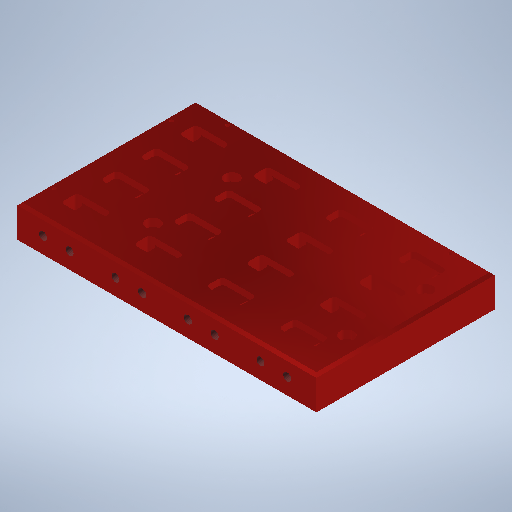
# Autodesk Inventor part: Chuck - 16-pocket
Saved by Autodesk Inventor 2025 (Build 290162000, 162)
## iProperties
Created: 2014-01-09
Part Number: Chuck - 16-pocket
Material: Aluminum, Anodized Red
Document SubType Name: Modeling
Designer: Caleb Fangmeier
Density: 2.7 g/cm^3
Project: CMS ETL
Mass: 2699.72 g
Surface Area: 1115.91 cm^2
Volume: 999.896 cm^3
Appearance: Anodized - Red
Author: Frank Meier
Autodesk Inventor part; units mm, degrees
ref_plane "YZ Plane" through (0, 0, 0) normal (1, 0, 0) x (0, 1, 0)
ref_plane "XZ Plane" through (0, 0, 0) normal (0, 1, 0) x (-1, 0, 0)
ref_plane "XY Plane" through (0, 0, 0) normal (0, 0, 1) x (1, 0, 0)
sketch "Skizze1" plane through (0, 0, 0) normal (0, 0, 1) x (1, 0, 0)
  line L0 (-117.5, -70) -> (117.5, -70)
  line L1 (117.5, -70) -> (117.5, 70)
  line L2 (117.5, 70) -> (-117.5, 70)
  line L3 (-117.5, 70) -> (-117.5, -70)
  line L4 (-117.5, -70) -> (117.5, 70) construction
  line L5 (117.5, -70) -> (-117.5, 70) construction
  point P0 (0, 0)
  dimension "d0" = 235
  dimension "d2" = 140
  constraints: 12 end point, 2 midpoint, 2 parallel, 1 horizontal, 1 perpendicular
  measures "d0" distance of L1.end L2.end
  measures "d2" distance of L0.end L1.end
extrude "Extrusion1" add sketch "Skizze1" along normal blind 25.4
chamfer "Fase1" distance 2 angle 45 4 edges at (0, -70, 25.4) (-117.5, 0, 25.4) (0, 70, 25.4) (117.5, 0, 25.4)
sketch "Alignment Holes" plane through (0, 0, 25.4) normal (0, 0, 1) x (1, 0, 0)
  line L0 (117.5, 70) -> (-117.5, 70) projected
  line L1 (117.5, -70) -> (117.5, 70) projected
  line L2 (-117.5, 70) -> (-117.5, -70) projected
  line L3 (-117.5, -70) -> (117.5, -70) projected
  point P0 (-112.5, 46)
  point P1 (-112.5, -46)
  point P2 (-87.5, 65)
  point P3 (87.5, 65)
  dimension "d153" = 24
  dimension "d154" = 24
  dimension "d155" = 5
  dimension "d158" = 5
  dimension "d159" = 5
  dimension "d160" = 30
  dimension "d161" = 30
  dimension "d162" = 5
  measures "d153" distance from line of L0 point (-112.5, 46)
  measures "d154" distance from line of L3 point (-112.5, -46)
  measures "d155" distance from line of L2 point (-112.5, -46)
  measures "d158" distance from line of L2 point (-112.5, 46)
  measures "d159" distance from line of L0 point (-87.5, 65)
  measures "d160" distance from line of L2 point (-87.5, 65)
  measures "d161" distance from line of L1 point (87.5, 65)
  measures "d162" distance from line of L0 point (87.5, 65)
hole "Bohrung7" at (-112.5, 46, 25.4) at (-112.5, -46, 25.4) at (-87.5, 65, 25.4) at (87.5, 65, 25.4) direction (0, 0, -1) diameter 3 end through all
sketch "Wells" plane through (0, 0, 25.4) normal (0, 0, 1) x (1, 0, 0)
  line L0 (-97.5, 53) -> (-76.5, 53)
  line L1 (-73.5, 50) -> (-73.5, 43)
  line L2 (-76.5, 40) -> (-97.5, 40)
  line L3 (-100.5, 43) -> (-100.5, 50)
  circle A0 centre (-87.5, 65) radius 1.5 projected
  circle A1 centre (-112.5, 46) radius 1.5 projected
  arc A2 (-97.5, 53) -> (-100.5, 50) centre (-97.5, 50) ccw
  arc A3 (-73.5, 50) -> (-76.5, 53) centre (-76.5, 50) ccw
  arc A4 (-76.5, 40) -> (-73.5, 43) centre (-76.5, 43) ccw
  arc A5 (-100.5, 43) -> (-97.5, 40) centre (-97.5, 43) ccw
  arc A6 (-40.5, 53) -> (-43.5, 50) centre (-40.5, 50) ccw
  line L4 (-43.5, 43) -> (-43.5, 50)
  arc A7 (-43.5, 43) -> (-40.5, 40) centre (-40.5, 43) ccw
  line L5 (-40.5, 53) -> (-19.5, 53)
  arc A8 (-16.5, 50) -> (-19.5, 53) centre (-19.5, 50) ccw
  line L6 (-16.5, 50) -> (-16.5, 43)
  line L7 (-19.5, 40) -> (-40.5, 40)
  arc A9 (-19.5, 40) -> (-16.5, 43) centre (-19.5, 43) ccw
  arc A10 (16.5, 53) -> (13.5, 50) centre (16.5, 50) ccw
  line L8 (13.5, 43) -> (13.5, 50)
  arc A11 (13.5, 43) -> (16.5, 40) centre (16.5, 43) ccw
  line L9 (16.5, 53) -> (37.5, 53)
  arc A12 (40.5, 50) -> (37.5, 53) centre (37.5, 50) ccw
  line L10 (40.5, 50) -> (40.5, 43)
  line L11 (37.5, 40) -> (16.5, 40)
  arc A13 (37.5, 40) -> (40.5, 43) centre (37.5, 43) ccw
  arc A14 (73.5, 53) -> (70.5, 50) centre (73.5, 50) ccw
  line L12 (70.5, 43) -> (70.5, 50)
  arc A15 (70.5, 43) -> (73.5, 40) centre (73.5, 43) ccw
  line L13 (73.5, 53) -> (94.5, 53)
  arc A16 (97.5, 50) -> (94.5, 53) centre (94.5, 50) ccw
  line L14 (97.5, 50) -> (97.5, 43)
  line L15 (94.5, 40) -> (73.5, 40)
  arc A17 (94.5, 40) -> (97.5, 43) centre (94.5, 43) ccw
  arc A18 (-97.5, 22) -> (-100.5, 19) centre (-97.5, 19) ccw
  line L16 (-100.5, 12) -> (-100.5, 19)
  arc A19 (-100.5, 12) -> (-97.5, 9) centre (-97.5, 12) ccw
  line L17 (-97.5, 22) -> (-76.5, 22)
  arc A20 (-73.5, 19) -> (-76.5, 22) centre (-76.5, 19) ccw
  line L18 (-73.5, 19) -> (-73.5, 12)
  line L19 (-76.5, 9) -> (-97.5, 9)
  arc A21 (-76.5, 9) -> (-73.5, 12) centre (-76.5, 12) ccw
  arc A22 (-40.5, 22) -> (-43.5, 19) centre (-40.5, 19) ccw
  line L20 (-43.5, 12) -> (-43.5, 19)
  arc A23 (-43.5, 12) -> (-40.5, 9) centre (-40.5, 12) ccw
  line L21 (-40.5, 22) -> (-19.5, 22)
  arc A24 (-16.5, 19) -> (-19.5, 22) centre (-19.5, 19) ccw
  line L22 (-16.5, 19) -> (-16.5, 12)
  line L23 (-19.5, 9) -> (-40.5, 9)
  arc A25 (-19.5, 9) -> (-16.5, 12) centre (-19.5, 12) ccw
  arc A26 (16.5, 22) -> (13.5, 19) centre (16.5, 19) ccw
  line L24 (13.5, 12) -> (13.5, 19)
  arc A27 (13.5, 12) -> (16.5, 9) centre (16.5, 12) ccw
  line L25 (16.5, 22) -> (37.5, 22)
  arc A28 (40.5, 19) -> (37.5, 22) centre (37.5, 19) ccw
  line L26 (40.5, 19) -> (40.5, 12)
  line L27 (37.5, 9) -> (16.5, 9)
  arc A29 (37.5, 9) -> (40.5, 12) centre (37.5, 12) ccw
  arc A30 (73.5, 22) -> (70.5, 19) centre (73.5, 19) ccw
  line L28 (70.5, 12) -> (70.5, 19)
  arc A31 (70.5, 12) -> (73.5, 9) centre (73.5, 12) ccw
  line L29 (73.5, 22) -> (94.5, 22)
  arc A32 (97.5, 19) -> (94.5, 22) centre (94.5, 19) ccw
  line L30 (97.5, 19) -> (97.5, 12)
  line L31 (94.5, 9) -> (73.5, 9)
  arc A33 (94.5, 9) -> (97.5, 12) centre (94.5, 12) ccw
  arc A34 (-97.5, -9) -> (-100.5, -12) centre (-97.5, -12) ccw
  line L32 (-100.5, -19) -> (-100.5, -12)
  arc A35 (-100.5, -19) -> (-97.5, -22) centre (-97.5, -19) ccw
  line L33 (-97.5, -9) -> (-76.5, -9)
  arc A36 (-73.5, -12) -> (-76.5, -9) centre (-76.5, -12) ccw
  line L34 (-73.5, -12) -> (-73.5, -19)
  line L35 (-76.5, -22) -> (-97.5, -22)
  arc A37 (-76.5, -22) -> (-73.5, -19) centre (-76.5, -19) ccw
  arc A38 (-40.5, -9) -> (-43.5, -12) centre (-40.5, -12) ccw
  line L36 (-43.5, -19) -> (-43.5, -12)
  arc A39 (-43.5, -19) -> (-40.5, -22) centre (-40.5, -19) ccw
  line L37 (-40.5, -9) -> (-19.5, -9)
  arc A40 (-16.5, -12) -> (-19.5, -9) centre (-19.5, -12) ccw
  line L38 (-16.5, -12) -> (-16.5, -19)
  line L39 (-19.5, -22) -> (-40.5, -22)
  arc A41 (-19.5, -22) -> (-16.5, -19) centre (-19.5, -19) ccw
  arc A42 (16.5, -9) -> (13.5, -12) centre (16.5, -12) ccw
  line L40 (13.5, -19) -> (13.5, -12)
  arc A43 (13.5, -19) -> (16.5, -22) centre (16.5, -19) ccw
  line L41 (16.5, -9) -> (37.5, -9)
  arc A44 (40.5, -12) -> (37.5, -9) centre (37.5, -12) ccw
  line L42 (40.5, -12) -> (40.5, -19)
  line L43 (37.5, -22) -> (16.5, -22)
  arc A45 (37.5, -22) -> (40.5, -19) centre (37.5, -19) ccw
  arc A46 (73.5, -9) -> (70.5, -12) centre (73.5, -12) ccw
  line L44 (70.5, -19) -> (70.5, -12)
  arc A47 (70.5, -19) -> (73.5, -22) centre (73.5, -19) ccw
  line L45 (73.5, -9) -> (94.5, -9)
  arc A48 (97.5, -12) -> (94.5, -9) centre (94.5, -12) ccw
  line L46 (97.5, -12) -> (97.5, -19)
  line L47 (94.5, -22) -> (73.5, -22)
  arc A49 (94.5, -22) -> (97.5, -19) centre (94.5, -19) ccw
  arc A50 (-97.5, -40) -> (-100.5, -43) centre (-97.5, -43) ccw
  line L48 (-100.5, -50) -> (-100.5, -43)
  arc A51 (-100.5, -50) -> (-97.5, -53) centre (-97.5, -50) ccw
  line L49 (-97.5, -40) -> (-76.5, -40)
  arc A52 (-73.5, -43) -> (-76.5, -40) centre (-76.5, -43) ccw
  line L50 (-73.5, -43) -> (-73.5, -50)
  line L51 (-76.5, -53) -> (-97.5, -53)
  arc A53 (-76.5, -53) -> (-73.5, -50) centre (-76.5, -50) ccw
  arc A54 (-40.5, -40) -> (-43.5, -43) centre (-40.5, -43) ccw
  line L52 (-43.5, -50) -> (-43.5, -43)
  arc A55 (-43.5, -50) -> (-40.5, -53) centre (-40.5, -50) ccw
  line L53 (-40.5, -40) -> (-19.5, -40)
  arc A56 (-16.5, -43) -> (-19.5, -40) centre (-19.5, -43) ccw
  line L54 (-16.5, -43) -> (-16.5, -50)
  line L55 (-19.5, -53) -> (-40.5, -53)
  arc A57 (-19.5, -53) -> (-16.5, -50) centre (-19.5, -50) ccw
  arc A58 (16.5, -40) -> (13.5, -43) centre (16.5, -43) ccw
  line L56 (13.5, -50) -> (13.5, -43)
  arc A59 (13.5, -50) -> (16.5, -53) centre (16.5, -50) ccw
  line L57 (16.5, -40) -> (37.5, -40)
  arc A60 (40.5, -43) -> (37.5, -40) centre (37.5, -43) ccw
  line L58 (40.5, -43) -> (40.5, -50)
  line L59 (37.5, -53) -> (16.5, -53)
  arc A61 (37.5, -53) -> (40.5, -50) centre (37.5, -50) ccw
  arc A62 (73.5, -40) -> (70.5, -43) centre (73.5, -43) ccw
  line L60 (70.5, -50) -> (70.5, -43)
  arc A63 (70.5, -50) -> (73.5, -53) centre (73.5, -50) ccw
  line L61 (73.5, -40) -> (94.5, -40)
  arc A64 (97.5, -43) -> (94.5, -40) centre (94.5, -43) ccw
  line L62 (97.5, -43) -> (97.5, -50)
  line L63 (94.5, -53) -> (73.5, -53)
  arc A65 (94.5, -53) -> (97.5, -50) centre (94.5, -50) ccw
  line L64 (117.5, 70) -> (-117.5, 70) projected
  line L65 (-117.5, 70) -> (-117.5, -70) projected
  line L66 (-117.5, -70) -> (117.5, -70) projected
  line L67 (117.5, -70) -> (117.5, 70) projected
  point P0 (0, 0)
  point P1 (-73.5, 40)
  point P2 (-73.5, 53)
  point P3 (-100.5, 40)
  point P4 (-43.5, 40)
  point P5 (-16.5, 53)
  point P6 (-16.5, 40)
  point P7 (13.5, 40)
  point P8 (40.5, 53)
  point P9 (40.5, 40)
  point P10 (70.5, 40)
  point P11 (97.5, 53)
  point P12 (97.5, 40)
  point P13 (-100.5, 9)
  point P14 (-73.5, 22)
  point P15 (-73.5, 9)
  point P16 (-43.5, 9)
  point P17 (-16.5, 22)
  point P18 (-16.5, 9)
  point P19 (13.5, 9)
  point P20 (40.5, 22)
  point P21 (40.5, 9)
  point P22 (70.5, 9)
  point P23 (97.5, 22)
  point P24 (97.5, 9)
  point P25 (-100.5, -22)
  point P26 (-73.5, -9)
  point P27 (-73.5, -22)
  point P28 (-43.5, -22)
  point P29 (-16.5, -9)
  point P30 (-16.5, -22)
  point P31 (13.5, -22)
  point P32 (40.5, -9)
  point P33 (40.5, -22)
  point P34 (70.5, -22)
  point P35 (97.5, -9)
  point P36 (97.5, -22)
  point P37 (-100.5, -53)
  point P38 (-73.5, -40)
  point P39 (-73.5, -53)
  point P40 (-43.5, -53)
  point P41 (-16.5, -40)
  point P42 (-16.5, -53)
  point P43 (13.5, -53)
  point P44 (40.5, -40)
  point P45 (40.5, -53)
  point P46 (70.5, -53)
  point P47 (97.5, -40)
  point P48 (97.5, -53)
  dimension "d259" = 27
  dimension "d260" = 13
  dimension "d266" = 3
  dimension "d269" = 57
  dimension "d272" = 31
  dimension "d476" = 17
  dimension "d477" = 17
  dimension "d478" = 17
  dimension "d479" = 20
  constraints: 128 end point, 128 point on circle, 96 point on line, 64 centre point, 8 tangent, 3 equal radius, 2 collinear, 2 horizontal, 2 parallel, 1 perpendicular, 1 vertical, 343 other
  measures "d259" distance of point (-73.5, 40) point (-100.5, 40)
  measures "d260" distance of point (-73.5, 53) point (-73.5, 40)
  measures "d266" radius of A2
  measures "d269" distance of L3.end L4.end
  measures "d272" distance of L3.end L16.end
  measures "d476" distance between parallel lines of L64 L0
  measures "d477" distance between parallel lines of L65 L3
  measures "d478" distance between parallel lines of L66 L51
  measures "d479" distance between parallel lines of L67 L14
extrude "Extrusion6" cut sketch "Wells" against normal blind 5 contours L0 A3 L1 A4 L2 A5 L3 A2 | L5 A8 L6 A9 L7 A7 L4 A6 | L9 A12 L10 A13 L11 A11 L8 A10 | L13 A16 L14 A17 L15 A15 L12 A14 | L17 A20 L18 A21 L19 A19 L16 A18 | L21 A24 L22 A25 L23 A23 L20 A22 | L25 A28 L26 A29 L27 A27 L24 A26 | L29 A32 L30 A33 L31 A31 L28 A30 | L33 A36 L34 A37 L35 A35 L32 A34 | L37 A40 L38 A41 L39 A39 L36 A38 | L41 A44 L42 A45 L43 A43 L40 A42 | L45 A48 L46 A49 L47 A47 L44 A46 | L49 A52 L50 A53 L51 A51 L48 A50 | L53 A56 L54 A57 L55 A55 L52 A54 | L57 A60 L58 A61 L59 A59 L56 A58 | L61 A64 L62 A65 L63 A63 L60 A62
sketch "Sketch22" plane through (0, 0, 25.4) normal (0, 0, 1) x (1, 0, 0)
  point P0 (0, 0)
  point P1 (102.4, -31)
  point P2 (-50, -31)
  point P3 (-50, 31)
  point P4 (102.4, 31)
  dimension "d383" = 152.4
  dimension "d384" = 31
  dimension "d385" = 62
  dimension "d503" = 50
  constraints: 2 horizontal alignment, 2 vertical alignment
  measures "d383" distance of point (102.4, -31) point (-50, -31)
  measures "d384" vertical distance of point (102.4, -31) point (0, 0)
  measures "d385" distance of point (102.4, -31) point (102.4, 31)
  measures "d503" horizontal distance of point (-50, 31) point (0, 0)
hole "Hole18" at (102.4, -31, 25.4) at (-50, -31, 25.4) at (-50, 31, 25.4) at (102.4, 31, 25.4) direction (0, 0, -1) diameter 6.528 end through all counterbore diameter 11.113 counterbore depth 6.35 clearance for "Socket Head Cap Screw" size "1/4" standard "Ansi Unified Screw Threads"
sketch "Sketch24" plane through (0, 0, 25.4) normal (0, 0, 1) x (1, 0, 0)
  line L0 (-76.5, 40) -> (-97.5, 40) projected
  arc A0 (-76.5, 40) -> (-73.5, 43) centre (-76.5, 43) ccw projected
  line L1 (-73.5, 50) -> (-73.5, 43) projected
  arc A1 (-73.5, 50) -> (-76.5, 53) centre (-76.5, 50) ccw projected
  line L2 (-97.5, 53) -> (-76.5, 53) projected
  arc A2 (-97.5, 53) -> (-100.5, 50) centre (-97.5, 50) ccw projected
  line L3 (-100.5, 43) -> (-100.5, 50) projected
  arc A3 (-100.5, 43) -> (-97.5, 40) centre (-97.5, 43) ccw projected
  line L4 (-76.5, 39.25) -> (-97.5, 39.25)
  line L5 (-101.25, 43) -> (-101.25, 50)
  line L6 (-97.5, 53.75) -> (-76.5, 53.75)
  line L7 (-72.75, 50) -> (-72.75, 43)
  line L8 (-76.5, 37.75) -> (-97.5, 37.75)
  line L9 (-102.75, 43) -> (-102.75, 50)
  line L10 (-97.5, 55.25) -> (-76.5, 55.25)
  line L11 (-71.25, 50) -> (-71.25, 43)
  arc A4 (-97.5, 53.75) -> (-101.25, 50) centre (-97.5, 50) ccw
  arc A5 (-97.5, 55.25) -> (-102.75, 50) centre (-97.5, 50) ccw
  arc A6 (-101.25, 43) -> (-97.5, 39.25) centre (-97.5, 43) ccw
  arc A7 (-76.5, 39.25) -> (-72.75, 43) centre (-76.5, 43) ccw
  arc A8 (-72.75, 50) -> (-76.5, 53.75) centre (-76.5, 50) ccw
  arc A9 (-102.75, 43) -> (-97.5, 37.75) centre (-97.5, 43) ccw
  arc A10 (-76.5, 37.75) -> (-71.25, 43) centre (-76.5, 43) ccw
  arc A11 (-71.25, 50) -> (-76.5, 55.25) centre (-76.5, 50) ccw
  arc A12 (-19.5, 39.25) -> (-15.75, 43) centre (-19.5, 43) ccw
  arc A13 (-19.5, 37.75) -> (-14.25, 43) centre (-19.5, 43) ccw
  arc A14 (-15.75, 50) -> (-19.5, 53.75) centre (-19.5, 50) ccw
  arc A15 (-14.25, 50) -> (-19.5, 55.25) centre (-19.5, 50) ccw
  line L12 (-14.25, 50) -> (-14.25, 43)
  line L13 (-15.75, 50) -> (-15.75, 43)
  line L14 (-19.5, 37.75) -> (-40.5, 37.75)
  line L15 (-19.5, 39.25) -> (-40.5, 39.25)
  line L16 (-40.5, 55.25) -> (-19.5, 55.25)
  line L17 (-40.5, 53.75) -> (-19.5, 53.75)
  line L18 (-44.25, 43) -> (-44.25, 50)
  line L19 (-45.75, 43) -> (-45.75, 50)
  arc A16 (-44.25, 43) -> (-40.5, 39.25) centre (-40.5, 43) ccw
  arc A17 (-45.75, 43) -> (-40.5, 37.75) centre (-40.5, 43) ccw
  arc A18 (-40.5, 53.75) -> (-44.25, 50) centre (-40.5, 50) ccw
  arc A19 (-40.5, 55.25) -> (-45.75, 50) centre (-40.5, 50) ccw
  arc A20 (37.5, 39.25) -> (41.25, 43) centre (37.5, 43) ccw
  arc A21 (37.5, 37.75) -> (42.75, 43) centre (37.5, 43) ccw
  arc A22 (41.25, 50) -> (37.5, 53.75) centre (37.5, 50) ccw
  arc A23 (42.75, 50) -> (37.5, 55.25) centre (37.5, 50) ccw
  line L20 (42.75, 50) -> (42.75, 43)
  line L21 (41.25, 50) -> (41.25, 43)
  line L22 (37.5, 37.75) -> (16.5, 37.75)
  line L23 (37.5, 39.25) -> (16.5, 39.25)
  line L24 (16.5, 55.25) -> (37.5, 55.25)
  line L25 (16.5, 53.75) -> (37.5, 53.75)
  line L26 (12.75, 43) -> (12.75, 50)
  line L27 (11.25, 43) -> (11.25, 50)
  arc A24 (12.75, 43) -> (16.5, 39.25) centre (16.5, 43) ccw
  arc A25 (11.25, 43) -> (16.5, 37.75) centre (16.5, 43) ccw
  arc A26 (16.5, 53.75) -> (12.75, 50) centre (16.5, 50) ccw
  arc A27 (16.5, 55.25) -> (11.25, 50) centre (16.5, 50) ccw
  arc A28 (94.5, 39.25) -> (98.25, 43) centre (94.5, 43) ccw
  arc A29 (94.5, 37.75) -> (99.75, 43) centre (94.5, 43) ccw
  arc A30 (98.25, 50) -> (94.5, 53.75) centre (94.5, 50) ccw
  arc A31 (99.75, 50) -> (94.5, 55.25) centre (94.5, 50) ccw
  line L28 (99.75, 50) -> (99.75, 43)
  line L29 (98.25, 50) -> (98.25, 43)
  line L30 (94.5, 37.75) -> (73.5, 37.75)
  line L31 (94.5, 39.25) -> (73.5, 39.25)
  line L32 (73.5, 55.25) -> (94.5, 55.25)
  line L33 (73.5, 53.75) -> (94.5, 53.75)
  line L34 (69.75, 43) -> (69.75, 50)
  line L35 (68.25, 43) -> (68.25, 50)
  arc A32 (69.75, 43) -> (73.5, 39.25) centre (73.5, 43) ccw
  arc A33 (68.25, 43) -> (73.5, 37.75) centre (73.5, 43) ccw
  arc A34 (73.5, 53.75) -> (69.75, 50) centre (73.5, 50) ccw
  arc A35 (73.5, 55.25) -> (68.25, 50) centre (73.5, 50) ccw
  arc A36 (-76.5, 8.25) -> (-72.75, 12) centre (-76.5, 12) ccw
  arc A37 (-76.5, 6.75) -> (-71.25, 12) centre (-76.5, 12) ccw
  arc A38 (-72.75, 19) -> (-76.5, 22.75) centre (-76.5, 19) ccw
  arc A39 (-71.25, 19) -> (-76.5, 24.25) centre (-76.5, 19) ccw
  line L36 (-71.25, 19) -> (-71.25, 12)
  line L37 (-72.75, 19) -> (-72.75, 12)
  line L38 (-76.5, 6.75) -> (-97.5, 6.75)
  line L39 (-76.5, 8.25) -> (-97.5, 8.25)
  line L40 (-97.5, 24.25) -> (-76.5, 24.25)
  line L41 (-97.5, 22.75) -> (-76.5, 22.75)
  line L42 (-101.25, 12) -> (-101.25, 19)
  line L43 (-102.75, 12) -> (-102.75, 19)
  arc A40 (-101.25, 12) -> (-97.5, 8.25) centre (-97.5, 12) ccw
  arc A41 (-102.75, 12) -> (-97.5, 6.75) centre (-97.5, 12) ccw
  arc A42 (-97.5, 22.75) -> (-101.25, 19) centre (-97.5, 19) ccw
  arc A43 (-97.5, 24.25) -> (-102.75, 19) centre (-97.5, 19) ccw
  arc A44 (-19.5, 8.25) -> (-15.75, 12) centre (-19.5, 12) ccw
  arc A45 (-19.5, 6.75) -> (-14.25, 12) centre (-19.5, 12) ccw
  arc A46 (-15.75, 19) -> (-19.5, 22.75) centre (-19.5, 19) ccw
  arc A47 (-14.25, 19) -> (-19.5, 24.25) centre (-19.5, 19) ccw
  line L44 (-14.25, 19) -> (-14.25, 12)
  line L45 (-15.75, 19) -> (-15.75, 12)
  line L46 (-19.5, 6.75) -> (-40.5, 6.75)
  line L47 (-19.5, 8.25) -> (-40.5, 8.25)
  line L48 (-40.5, 24.25) -> (-19.5, 24.25)
  line L49 (-40.5, 22.75) -> (-19.5, 22.75)
  line L50 (-44.25, 12) -> (-44.25, 19)
  line L51 (-45.75, 12) -> (-45.75, 19)
  arc A48 (-44.25, 12) -> (-40.5, 8.25) centre (-40.5, 12) ccw
  arc A49 (-45.75, 12) -> (-40.5, 6.75) centre (-40.5, 12) ccw
  arc A50 (-40.5, 22.75) -> (-44.25, 19) centre (-40.5, 19) ccw
  arc A51 (-40.5, 24.25) -> (-45.75, 19) centre (-40.5, 19) ccw
  arc A52 (37.5, 8.25) -> (41.25, 12) centre (37.5, 12) ccw
  arc A53 (37.5, 6.75) -> (42.75, 12) centre (37.5, 12) ccw
  arc A54 (41.25, 19) -> (37.5, 22.75) centre (37.5, 19) ccw
  arc A55 (42.75, 19) -> (37.5, 24.25) centre (37.5, 19) ccw
  line L52 (42.75, 19) -> (42.75, 12)
  line L53 (41.25, 19) -> (41.25, 12)
  line L54 (37.5, 6.75) -> (16.5, 6.75)
  line L55 (37.5, 8.25) -> (16.5, 8.25)
  line L56 (16.5, 24.25) -> (37.5, 24.25)
  line L57 (16.5, 22.75) -> (37.5, 22.75)
  line L58 (12.75, 12) -> (12.75, 19)
  line L59 (11.25, 12) -> (11.25, 19)
  arc A56 (12.75, 12) -> (16.5, 8.25) centre (16.5, 12) ccw
  arc A57 (11.25, 12) -> (16.5, 6.75) centre (16.5, 12) ccw
  arc A58 (16.5, 22.75) -> (12.75, 19) centre (16.5, 19) ccw
  arc A59 (16.5, 24.25) -> (11.25, 19) centre (16.5, 19) ccw
  arc A60 (94.5, 8.25) -> (98.25, 12) centre (94.5, 12) ccw
  arc A61 (94.5, 6.75) -> (99.75, 12) centre (94.5, 12) ccw
  arc A62 (98.25, 19) -> (94.5, 22.75) centre (94.5, 19) ccw
  arc A63 (99.75, 19) -> (94.5, 24.25) centre (94.5, 19) ccw
  line L60 (99.75, 19) -> (99.75, 12)
  line L61 (98.25, 19) -> (98.25, 12)
  line L62 (94.5, 6.75) -> (73.5, 6.75)
  line L63 (94.5, 8.25) -> (73.5, 8.25)
  line L64 (73.5, 24.25) -> (94.5, 24.25)
  line L65 (73.5, 22.75) -> (94.5, 22.75)
  line L66 (69.75, 12) -> (69.75, 19)
  line L67 (68.25, 12) -> (68.25, 19)
  arc A64 (69.75, 12) -> (73.5, 8.25) centre (73.5, 12) ccw
  arc A65 (68.25, 12) -> (73.5, 6.75) centre (73.5, 12) ccw
  arc A66 (73.5, 22.75) -> (69.75, 19) centre (73.5, 19) ccw
  arc A67 (73.5, 24.25) -> (68.25, 19) centre (73.5, 19) ccw
  arc A68 (-76.5, -22.75) -> (-72.75, -19) centre (-76.5, -19) ccw
  arc A69 (-76.5, -24.25) -> (-71.25, -19) centre (-76.5, -19) ccw
  arc A70 (-72.75, -12) -> (-76.5, -8.25) centre (-76.5, -12) ccw
  arc A71 (-71.25, -12) -> (-76.5, -6.75) centre (-76.5, -12) ccw
  line L68 (-71.25, -12) -> (-71.25, -19)
  line L69 (-72.75, -12) -> (-72.75, -19)
  line L70 (-76.5, -24.25) -> (-97.5, -24.25)
  line L71 (-76.5, -22.75) -> (-97.5, -22.75)
  line L72 (-97.5, -6.75) -> (-76.5, -6.75)
  line L73 (-97.5, -8.25) -> (-76.5, -8.25)
  line L74 (-101.25, -19) -> (-101.25, -12)
  line L75 (-102.75, -19) -> (-102.75, -12)
  arc A72 (-101.25, -19) -> (-97.5, -22.75) centre (-97.5, -19) ccw
  arc A73 (-102.75, -19) -> (-97.5, -24.25) centre (-97.5, -19) ccw
  arc A74 (-97.5, -8.25) -> (-101.25, -12) centre (-97.5, -12) ccw
  arc A75 (-97.5, -6.75) -> (-102.75, -12) centre (-97.5, -12) ccw
  arc A76 (-19.5, -22.75) -> (-15.75, -19) centre (-19.5, -19) ccw
  arc A77 (-19.5, -24.25) -> (-14.25, -19) centre (-19.5, -19) ccw
  arc A78 (-15.75, -12) -> (-19.5, -8.25) centre (-19.5, -12) ccw
  arc A79 (-14.25, -12) -> (-19.5, -6.75) centre (-19.5, -12) ccw
  line L76 (-14.25, -12) -> (-14.25, -19)
  line L77 (-15.75, -12) -> (-15.75, -19)
  line L78 (-19.5, -24.25) -> (-40.5, -24.25)
  line L79 (-19.5, -22.75) -> (-40.5, -22.75)
  line L80 (-40.5, -6.75) -> (-19.5, -6.75)
  line L81 (-40.5, -8.25) -> (-19.5, -8.25)
  line L82 (-44.25, -19) -> (-44.25, -12)
  line L83 (-45.75, -19) -> (-45.75, -12)
  arc A80 (-44.25, -19) -> (-40.5, -22.75) centre (-40.5, -19) ccw
  arc A81 (-45.75, -19) -> (-40.5, -24.25) centre (-40.5, -19) ccw
  arc A82 (-40.5, -8.25) -> (-44.25, -12) centre (-40.5, -12) ccw
  arc A83 (-40.5, -6.75) -> (-45.75, -12) centre (-40.5, -12) ccw
  arc A84 (37.5, -22.75) -> (41.25, -19) centre (37.5, -19) ccw
  arc A85 (37.5, -24.25) -> (42.75, -19) centre (37.5, -19) ccw
  arc A86 (41.25, -12) -> (37.5, -8.25) centre (37.5, -12) ccw
  arc A87 (42.75, -12) -> (37.5, -6.75) centre (37.5, -12) ccw
  line L84 (42.75, -12) -> (42.75, -19)
  line L85 (41.25, -12) -> (41.25, -19)
  line L86 (37.5, -24.25) -> (16.5, -24.25)
  line L87 (37.5, -22.75) -> (16.5, -22.75)
  line L88 (16.5, -6.75) -> (37.5, -6.75)
  line L89 (16.5, -8.25) -> (37.5, -8.25)
  line L90 (12.75, -19) -> (12.75, -12)
  line L91 (11.25, -19) -> (11.25, -12)
  arc A88 (12.75, -19) -> (16.5, -22.75) centre (16.5, -19) ccw
  arc A89 (11.25, -19) -> (16.5, -24.25) centre (16.5, -19) ccw
  arc A90 (16.5, -8.25) -> (12.75, -12) centre (16.5, -12) ccw
  arc A91 (16.5, -6.75) -> (11.25, -12) centre (16.5, -12) ccw
  arc A92 (94.5, -22.75) -> (98.25, -19) centre (94.5, -19) ccw
  arc A93 (94.5, -24.25) -> (99.75, -19) centre (94.5, -19) ccw
  arc A94 (98.25, -12) -> (94.5, -8.25) centre (94.5, -12) ccw
  arc A95 (99.75, -12) -> (94.5, -6.75) centre (94.5, -12) ccw
  line L92 (99.75, -12) -> (99.75, -19)
  line L93 (98.25, -12) -> (98.25, -19)
  line L94 (94.5, -24.25) -> (73.5, -24.25)
  line L95 (94.5, -22.75) -> (73.5, -22.75)
  line L96 (73.5, -6.75) -> (94.5, -6.75)
  line L97 (73.5, -8.25) -> (94.5, -8.25)
  line L98 (69.75, -19) -> (69.75, -12)
  line L99 (68.25, -19) -> (68.25, -12)
  arc A96 (69.75, -19) -> (73.5, -22.75) centre (73.5, -19) ccw
  arc A97 (68.25, -19) -> (73.5, -24.25) centre (73.5, -19) ccw
  arc A98 (73.5, -8.25) -> (69.75, -12) centre (73.5, -12) ccw
  arc A99 (73.5, -6.75) -> (68.25, -12) centre (73.5, -12) ccw
  arc A100 (-76.5, -53.75) -> (-72.75, -50) centre (-76.5, -50) ccw
  arc A101 (-76.5, -55.25) -> (-71.25, -50) centre (-76.5, -50) ccw
  arc A102 (-72.75, -43) -> (-76.5, -39.25) centre (-76.5, -43) ccw
  arc A103 (-71.25, -43) -> (-76.5, -37.75) centre (-76.5, -43) ccw
  line L100 (-71.25, -43) -> (-71.25, -50)
  line L101 (-72.75, -43) -> (-72.75, -50)
  line L102 (-76.5, -55.25) -> (-97.5, -55.25)
  line L103 (-76.5, -53.75) -> (-97.5, -53.75)
  line L104 (-97.5, -37.75) -> (-76.5, -37.75)
  line L105 (-97.5, -39.25) -> (-76.5, -39.25)
  line L106 (-101.25, -50) -> (-101.25, -43)
  line L107 (-102.75, -50) -> (-102.75, -43)
  arc A104 (-101.25, -50) -> (-97.5, -53.75) centre (-97.5, -50) ccw
  arc A105 (-102.75, -50) -> (-97.5, -55.25) centre (-97.5, -50) ccw
  arc A106 (-97.5, -39.25) -> (-101.25, -43) centre (-97.5, -43) ccw
  arc A107 (-97.5, -37.75) -> (-102.75, -43) centre (-97.5, -43) ccw
  arc A108 (-19.5, -53.75) -> (-15.75, -50) centre (-19.5, -50) ccw
  arc A109 (-19.5, -55.25) -> (-14.25, -50) centre (-19.5, -50) ccw
  arc A110 (-15.75, -43) -> (-19.5, -39.25) centre (-19.5, -43) ccw
  arc A111 (-14.25, -43) -> (-19.5, -37.75) centre (-19.5, -43) ccw
  line L108 (-14.25, -43) -> (-14.25, -50)
  line L109 (-15.75, -43) -> (-15.75, -50)
  line L110 (-19.5, -55.25) -> (-40.5, -55.25)
  line L111 (-19.5, -53.75) -> (-40.5, -53.75)
  line L112 (-40.5, -37.75) -> (-19.5, -37.75)
  line L113 (-40.5, -39.25) -> (-19.5, -39.25)
  line L114 (-44.25, -50) -> (-44.25, -43)
  line L115 (-45.75, -50) -> (-45.75, -43)
  arc A112 (-44.25, -50) -> (-40.5, -53.75) centre (-40.5, -50) ccw
  arc A113 (-45.75, -50) -> (-40.5, -55.25) centre (-40.5, -50) ccw
  arc A114 (-40.5, -39.25) -> (-44.25, -43) centre (-40.5, -43) ccw
  arc A115 (-40.5, -37.75) -> (-45.75, -43) centre (-40.5, -43) ccw
  arc A116 (37.5, -53.75) -> (41.25, -50) centre (37.5, -50) ccw
  arc A117 (37.5, -55.25) -> (42.75, -50) centre (37.5, -50) ccw
  arc A118 (41.25, -43) -> (37.5, -39.25) centre (37.5, -43) ccw
  arc A119 (42.75, -43) -> (37.5, -37.75) centre (37.5, -43) ccw
  line L116 (42.75, -43) -> (42.75, -50)
  line L117 (41.25, -43) -> (41.25, -50)
  line L118 (37.5, -55.25) -> (16.5, -55.25)
  line L119 (37.5, -53.75) -> (16.5, -53.75)
  line L120 (16.5, -37.75) -> (37.5, -37.75)
  line L121 (16.5, -39.25) -> (37.5, -39.25)
  line L122 (12.75, -50) -> (12.75, -43)
  line L123 (11.25, -50) -> (11.25, -43)
  arc A120 (12.75, -50) -> (16.5, -53.75) centre (16.5, -50) ccw
  arc A121 (11.25, -50) -> (16.5, -55.25) centre (16.5, -50) ccw
  arc A122 (16.5, -39.25) -> (12.75, -43) centre (16.5, -43) ccw
  arc A123 (16.5, -37.75) -> (11.25, -43) centre (16.5, -43) ccw
  arc A124 (94.5, -53.75) -> (98.25, -50) centre (94.5, -50) ccw
  arc A125 (94.5, -55.25) -> (99.75, -50) centre (94.5, -50) ccw
  arc A126 (98.25, -43) -> (94.5, -39.25) centre (94.5, -43) ccw
  arc A127 (99.75, -43) -> (94.5, -37.75) centre (94.5, -43) ccw
  line L124 (99.75, -43) -> (99.75, -50)
  line L125 (98.25, -43) -> (98.25, -50)
  line L126 (94.5, -55.25) -> (73.5, -55.25)
  line L127 (94.5, -53.75) -> (73.5, -53.75)
  line L128 (73.5, -37.75) -> (94.5, -37.75)
  line L129 (73.5, -39.25) -> (94.5, -39.25)
  line L130 (69.75, -50) -> (69.75, -43)
  line L131 (68.25, -50) -> (68.25, -43)
  arc A128 (69.75, -50) -> (73.5, -53.75) centre (73.5, -50) ccw
  arc A129 (68.25, -50) -> (73.5, -55.25) centre (73.5, -50) ccw
  arc A130 (73.5, -39.25) -> (69.75, -43) centre (73.5, -43) ccw
  arc A131 (73.5, -37.75) -> (68.25, -43) centre (73.5, -43) ccw
  point P0 (0, 0)
  dimension "d480" = 0.75
  dimension "d481" = 0.75
  dimension "d482" = 0.75
  dimension "d483" = 0.75
  dimension "d484" = 1.5
  dimension "d485" = 1.5
  dimension "d486" = 1.5
  dimension "d487" = 1.5
  dimension "d488" = 3
  dimension "d489" = 3.75
  dimension "d490" = 5.25
  dimension "d491" = 3.75
  dimension "d492" = 5.25
  dimension "d495" = 57
  dimension "d498" = 31
  constraints: 256 end point, 256 point on circle, 128 centre point, 16 tangent, 4 equal radius, 4 parallel, 3 horizontal, 2 perpendicular, 1 vertical, 600 other
  measures "d480" distance between parallel lines of L6 L2
  measures "d481" distance between parallel lines of L5 L3
  measures "d482" distance between parallel lines of L1 L7
  measures "d483" distance between parallel lines of L0 L4
  measures "d484" distance between parallel lines of L6 L10
  measures "d485" distance between parallel lines of L9 L5
  measures "d486" distance between parallel lines of L7 L11
  measures "d487" distance between parallel lines of L4 L8
  measures "d488" radius of A2
  measures "d489" radius of A4
  measures "d490" radius of A5
  measures "d491" radius of A6
  measures "d492" radius of A9
  measures "d495" distance of A7.centre A12.centre
  measures "d498" distance of A7.centre A36.centre
extrude "Extrusion10" [suppressed]
sketch "Sketch25" plane through (-117.5, -70, 0) normal (0, -1, 0) x (1, 0, 0)
  line L0 (233, 25.4) -> (2, 25.4) projected
  line L1 (0, 0) -> (235, 0) projected
  line L2 (0, 0) -> (0, 23.4) projected
  point P0 (117.5, 0)
  point P1 (20, 12.7)
  point P2 (41, 12.7)
  point P3 (98, 12.7)
  point P4 (77, 12.7)
  point P5 (155, 12.7)
  point P6 (134, 12.7)
  point P7 (212, 12.7)
  point P8 (191, 12.7)
  dimension "d504" = 25.4
  dimension "d505" = 12.7
  dimension "d506" = 21
  dimension "d507" = 20
  dimension "d510" = 57
  constraints: 1 horizontal, 1 horizontal alignment, 6 other
  measures "d504" distance between parallel lines of L0 L1
  measures "d505" distance from line of L1 point (20, 12.7)
  measures "d506" distance of point (20, 12.7) point (41, 12.7)
  measures "d507" distance from line of L2 point (20, 12.7)
  measures "d510" distance of point (41, 12.7) point (98, 12.7)
hole "Hole19" at (-97.5, -70, 12.7) at (-40.5, -70, 12.7) at (37.5, -70, 12.7) at (94.5, -70, 12.7) direction (0, 1, 0) diameter 5.9436 depth 28 tip angle 118 taper from width 6.3893 to width 5.9591 over 6.8859 thread size "1/16" designation "1/16 - 27 NPT" standard "NPT"
sketch "Sketch26" plane through (0, 0, 20.4) normal (0, 0, 1) x (1, 0, 0)
  line L0 (-76.5, 40) -> (-97.5, 40) projected
  arc A0 (-76.5, 40) -> (-73.5, 43) centre (-76.5, 43) ccw projected
  line L1 (-73.5, 50) -> (-73.5, 43) projected
  arc A1 (-73.5, 50) -> (-76.5, 53) centre (-76.5, 50) ccw projected
  line L2 (-97.5, 53) -> (-76.5, 53) projected
  arc A2 (-97.5, 53) -> (-100.5, 50) centre (-97.5, 50) ccw projected
  line L3 (-100.5, 43) -> (-100.5, 50) projected
  arc A3 (-100.5, 43) -> (-97.5, 40) centre (-97.5, 43) ccw projected
  line L4 (-97.5, 22) -> (-76.5, 22) projected
  arc A4 (-97.5, 22) -> (-100.5, 19) centre (-97.5, 19) ccw projected
  line L5 (-100.5, 12) -> (-100.5, 19) projected
  arc A5 (-100.5, 12) -> (-97.5, 9) centre (-97.5, 12) ccw projected
  line L6 (-76.5, 9) -> (-97.5, 9) projected
  arc A6 (-76.5, 9) -> (-73.5, 12) centre (-76.5, 12) ccw projected
  line L7 (-73.5, 19) -> (-73.5, 12) projected
  arc A7 (-73.5, 19) -> (-76.5, 22) centre (-76.5, 19) ccw projected
  line L8 (-97.5, -9) -> (-76.5, -9) projected
  arc A8 (-97.5, -9) -> (-100.5, -12) centre (-97.5, -12) ccw projected
  line L9 (-100.5, -19) -> (-100.5, -12) projected
  arc A9 (-100.5, -19) -> (-97.5, -22) centre (-97.5, -19) ccw projected
  line L10 (-76.5, -22) -> (-97.5, -22) projected
  arc A10 (-76.5, -22) -> (-73.5, -19) centre (-76.5, -19) ccw projected
  line L11 (-73.5, -12) -> (-73.5, -19) projected
  arc A11 (-73.5, -12) -> (-76.5, -9) centre (-76.5, -12) ccw projected
  line L12 (-97.5, -40) -> (-76.5, -40) projected
  arc A12 (-97.5, -40) -> (-100.5, -43) centre (-97.5, -43) ccw projected
  line L13 (-100.5, -50) -> (-100.5, -43) projected
  arc A13 (-100.5, -50) -> (-97.5, -53) centre (-97.5, -50) ccw projected
  line L14 (-76.5, -53) -> (-97.5, -53) projected
  arc A14 (-76.5, -53) -> (-73.5, -50) centre (-76.5, -50) ccw projected
  line L15 (-73.5, -43) -> (-73.5, -50) projected
  arc A15 (-73.5, -43) -> (-76.5, -40) centre (-76.5, -43) ccw projected
  line L16 (-40.5, -40) -> (-19.5, -40) projected
  arc A16 (-40.5, -40) -> (-43.5, -43) centre (-40.5, -43) ccw projected
  line L17 (-43.5, -50) -> (-43.5, -43) projected
  arc A17 (-43.5, -50) -> (-40.5, -53) centre (-40.5, -50) ccw projected
  line L18 (-19.5, -53) -> (-40.5, -53) projected
  arc A18 (-19.5, -53) -> (-16.5, -50) centre (-19.5, -50) ccw projected
  line L19 (-16.5, -43) -> (-16.5, -50) projected
  arc A19 (-16.5, -43) -> (-19.5, -40) centre (-19.5, -43) ccw projected
  line L20 (-40.5, -9) -> (-19.5, -9) projected
  arc A20 (-40.5, -9) -> (-43.5, -12) centre (-40.5, -12) ccw projected
  line L21 (-43.5, -19) -> (-43.5, -12) projected
  arc A21 (-43.5, -19) -> (-40.5, -22) centre (-40.5, -19) ccw projected
  line L22 (-19.5, -22) -> (-40.5, -22) projected
  arc A22 (-19.5, -22) -> (-16.5, -19) centre (-19.5, -19) ccw projected
  line L23 (-16.5, -12) -> (-16.5, -19) projected
  arc A23 (-16.5, -12) -> (-19.5, -9) centre (-19.5, -12) ccw projected
  line L24 (-40.5, 22) -> (-19.5, 22) projected
  arc A24 (-40.5, 22) -> (-43.5, 19) centre (-40.5, 19) ccw projected
  line L25 (-43.5, 12) -> (-43.5, 19) projected
  arc A25 (-43.5, 12) -> (-40.5, 9) centre (-40.5, 12) ccw projected
  line L26 (-19.5, 9) -> (-40.5, 9) projected
  arc A26 (-19.5, 9) -> (-16.5, 12) centre (-19.5, 12) ccw projected
  line L27 (-16.5, 19) -> (-16.5, 12) projected
  arc A27 (-16.5, 19) -> (-19.5, 22) centre (-19.5, 19) ccw projected
  line L28 (-40.5, 53) -> (-19.5, 53) projected
  arc A28 (-40.5, 53) -> (-43.5, 50) centre (-40.5, 50) ccw projected
  line L29 (-43.5, 43) -> (-43.5, 50) projected
  arc A29 (-43.5, 43) -> (-40.5, 40) centre (-40.5, 43) ccw projected
  line L30 (-19.5, 40) -> (-40.5, 40) projected
  arc A30 (-19.5, 40) -> (-16.5, 43) centre (-19.5, 43) ccw projected
  line L31 (-16.5, 50) -> (-16.5, 43) projected
  arc A31 (-16.5, 50) -> (-19.5, 53) centre (-19.5, 50) ccw projected
  line L32 (16.5, 53) -> (37.5, 53) projected
  arc A32 (16.5, 53) -> (13.5, 50) centre (16.5, 50) ccw projected
  line L33 (13.5, 43) -> (13.5, 50) projected
  arc A33 (13.5, 43) -> (16.5, 40) centre (16.5, 43) ccw projected
  line L34 (37.5, 40) -> (16.5, 40) projected
  arc A34 (37.5, 40) -> (40.5, 43) centre (37.5, 43) ccw projected
  line L35 (40.5, 50) -> (40.5, 43) projected
  arc A35 (40.5, 50) -> (37.5, 53) centre (37.5, 50) ccw projected
  line L36 (16.5, 22) -> (37.5, 22) projected
  arc A36 (16.5, 22) -> (13.5, 19) centre (16.5, 19) ccw projected
  line L37 (13.5, 12) -> (13.5, 19) projected
  arc A37 (13.5, 12) -> (16.5, 9) centre (16.5, 12) ccw projected
  line L38 (37.5, 9) -> (16.5, 9) projected
  arc A38 (37.5, 9) -> (40.5, 12) centre (37.5, 12) ccw projected
  line L39 (40.5, 19) -> (40.5, 12) projected
  arc A39 (40.5, 19) -> (37.5, 22) centre (37.5, 19) ccw projected
  line L40 (16.5, -9) -> (37.5, -9) projected
  arc A40 (16.5, -9) -> (13.5, -12) centre (16.5, -12) ccw projected
  line L41 (13.5, -19) -> (13.5, -12) projected
  arc A41 (13.5, -19) -> (16.5, -22) centre (16.5, -19) ccw projected
  line L42 (37.5, -22) -> (16.5, -22) projected
  arc A42 (37.5, -22) -> (40.5, -19) centre (37.5, -19) ccw projected
  line L43 (40.5, -12) -> (40.5, -19) projected
  arc A43 (40.5, -12) -> (37.5, -9) centre (37.5, -12) ccw projected
  line L44 (16.5, -40) -> (37.5, -40) projected
  arc A44 (16.5, -40) -> (13.5, -43) centre (16.5, -43) ccw projected
  line L45 (13.5, -50) -> (13.5, -43) projected
  arc A45 (13.5, -50) -> (16.5, -53) centre (16.5, -50) ccw projected
  line L46 (37.5, -53) -> (16.5, -53) projected
  arc A46 (37.5, -53) -> (40.5, -50) centre (37.5, -50) ccw projected
  line L47 (40.5, -43) -> (40.5, -50) projected
  arc A47 (40.5, -43) -> (37.5, -40) centre (37.5, -43) ccw projected
  line L48 (73.5, -40) -> (94.5, -40) projected
  arc A48 (73.5, -40) -> (70.5, -43) centre (73.5, -43) ccw projected
  line L49 (70.5, -50) -> (70.5, -43) projected
  arc A49 (70.5, -50) -> (73.5, -53) centre (73.5, -50) ccw projected
  line L50 (94.5, -53) -> (73.5, -53) projected
  arc A50 (94.5, -53) -> (97.5, -50) centre (94.5, -50) ccw projected
  line L51 (97.5, -43) -> (97.5, -50) projected
  arc A51 (97.5, -43) -> (94.5, -40) centre (94.5, -43) ccw projected
  line L52 (73.5, -9) -> (94.5, -9) projected
  arc A52 (73.5, -9) -> (70.5, -12) centre (73.5, -12) ccw projected
  line L53 (70.5, -19) -> (70.5, -12) projected
  arc A53 (70.5, -19) -> (73.5, -22) centre (73.5, -19) ccw projected
  line L54 (94.5, -22) -> (73.5, -22) projected
  arc A54 (94.5, -22) -> (97.5, -19) centre (94.5, -19) ccw projected
  line L55 (97.5, -12) -> (97.5, -19) projected
  arc A55 (97.5, -12) -> (94.5, -9) centre (94.5, -12) ccw projected
  line L56 (73.5, 22) -> (94.5, 22) projected
  arc A56 (73.5, 22) -> (70.5, 19) centre (73.5, 19) ccw projected
  line L57 (70.5, 12) -> (70.5, 19) projected
  arc A57 (70.5, 12) -> (73.5, 9) centre (73.5, 12) ccw projected
  line L58 (94.5, 9) -> (73.5, 9) projected
  arc A58 (94.5, 9) -> (97.5, 12) centre (94.5, 12) ccw projected
  line L59 (97.5, 19) -> (97.5, 12) projected
  arc A59 (97.5, 19) -> (94.5, 22) centre (94.5, 19) ccw projected
  line L60 (73.5, 53) -> (94.5, 53) projected
  arc A60 (73.5, 53) -> (70.5, 50) centre (73.5, 50) ccw projected
  line L61 (70.5, 43) -> (70.5, 50) projected
  arc A61 (70.5, 43) -> (73.5, 40) centre (73.5, 43) ccw projected
  line L62 (94.5, 40) -> (73.5, 40) projected
  arc A62 (94.5, 40) -> (97.5, 43) centre (94.5, 43) ccw projected
  line L63 (97.5, 50) -> (97.5, 43) projected
  arc A63 (97.5, 50) -> (94.5, 53) centre (94.5, 50) ccw projected
  line L64 (-40.5, -43) -> (-40.5, -50) construction
  line L65 (-37.5, -43) -> (-37.5, -50)
  line L66 (-43.5, -50) -> (-43.5, -43)
  arc A64 (-37.5, -43) -> (-43.5, -43) centre (-40.5, -43) ccw
  arc A65 (-43.5, -50) -> (-37.5, -50) centre (-40.5, -50) ccw
  line L67 (-19.5, -19) -> (-19.5, -12) construction
  line L68 (-22.5, -19) -> (-22.5, -12)
  line L69 (-16.5, -12) -> (-16.5, -19)
  arc A66 (-22.5, -19) -> (-16.5, -19) centre (-19.5, -19) ccw
  arc A67 (-16.5, -12) -> (-22.5, -12) centre (-19.5, -12) ccw
  line L70 (-97.5, -50) -> (-97.5, -43) construction
  line L71 (-94.5, -50) -> (-94.5, -43)
  line L72 (-100.5, -43) -> (-100.5, -50)
  arc A68 (-100.5, -50) -> (-94.5, -50) centre (-97.5, -50) ccw
  arc A69 (-94.5, -43) -> (-100.5, -43) centre (-97.5, -43) ccw
  line L73 (-76.5, -19) -> (-76.5, -12) construction
  line L74 (-79.5, -19) -> (-79.5, -12)
  line L75 (-73.5, -12) -> (-73.5, -19)
  arc A70 (-79.5, -19) -> (-73.5, -19) centre (-76.5, -19) ccw
  arc A71 (-73.5, -12) -> (-79.5, -12) centre (-76.5, -12) ccw
  line L76 (-97.5, 50) -> (-97.5, 43) construction
  line L77 (-94.5, 50) -> (-94.5, 43)
  line L78 (-100.5, 43) -> (-100.5, 50)
  arc A72 (-94.5, 50) -> (-100.5, 50) centre (-97.5, 50) ccw
  arc A73 (-100.5, 43) -> (-94.5, 43) centre (-97.5, 43) ccw
  line L79 (-76.5, 19) -> (-76.5, 12) construction
  line L80 (-79.5, 19) -> (-79.5, 12)
  line L81 (-73.5, 12) -> (-73.5, 19)
  arc A74 (-73.5, 19) -> (-79.5, 19) centre (-76.5, 19) ccw
  arc A75 (-79.5, 12) -> (-73.5, 12) centre (-76.5, 12) ccw
  line L82 (-19.5, 12) -> (-19.5, 19) construction
  line L83 (-22.5, 12) -> (-22.5, 19)
  line L84 (-16.5, 19) -> (-16.5, 12)
  arc A76 (-22.5, 12) -> (-16.5, 12) centre (-19.5, 12) ccw
  arc A77 (-16.5, 19) -> (-22.5, 19) centre (-19.5, 19) ccw
  line L85 (-40.5, 43) -> (-40.5, 50) construction
  line L86 (-37.5, 43) -> (-37.5, 50)
  line L87 (-43.5, 50) -> (-43.5, 43)
  arc A78 (-43.5, 43) -> (-37.5, 43) centre (-40.5, 43) ccw
  arc A79 (-37.5, 50) -> (-43.5, 50) centre (-40.5, 50) ccw
  line L88 (94.5, -50) -> (94.5, -43) construction
  line L89 (97.5, -50) -> (97.5, -43)
  line L90 (91.5, -43) -> (91.5, -50)
  arc A80 (91.5, -50) -> (97.5, -50) centre (94.5, -50) ccw
  arc A81 (97.5, -43) -> (91.5, -43) centre (94.5, -43) ccw
  line L91 (73.5, -19) -> (73.5, -12) construction
  line L92 (76.5, -19) -> (76.5, -12)
  line L93 (70.5, -12) -> (70.5, -19)
  arc A82 (70.5, -19) -> (76.5, -19) centre (73.5, -19) ccw
  arc A83 (76.5, -12) -> (70.5, -12) centre (73.5, -12) ccw
  line L94 (73.5, 12) -> (73.5, 19) construction
  line L95 (76.5, 12) -> (76.5, 19)
  line L96 (70.5, 19) -> (70.5, 12)
  arc A84 (70.5, 12) -> (76.5, 12) centre (73.5, 12) ccw
  arc A85 (76.5, 19) -> (70.5, 19) centre (73.5, 19) ccw
  line L97 (94.5, 43) -> (94.5, 50) construction
  line L98 (91.5, 43) -> (91.5, 50)
  line L99 (97.5, 50) -> (97.5, 43)
  arc A86 (91.5, 43) -> (97.5, 43) centre (94.5, 43) ccw
  arc A87 (97.5, 50) -> (91.5, 50) centre (94.5, 50) ccw
  line L100 (37.5, -50) -> (37.5, -43) construction
  line L101 (34.5, -50) -> (34.5, -43)
  line L102 (40.5, -43) -> (40.5, -50)
  arc A88 (34.5, -50) -> (40.5, -50) centre (37.5, -50) ccw
  arc A89 (40.5, -43) -> (34.5, -43) centre (37.5, -43) ccw
  line L103 (16.5, -19) -> (16.5, -12) construction
  line L104 (19.5, -19) -> (19.5, -12)
  line L105 (13.5, -12) -> (13.5, -19)
  arc A90 (13.5, -19) -> (19.5, -19) centre (16.5, -19) ccw
  arc A91 (19.5, -12) -> (13.5, -12) centre (16.5, -12) ccw
  line L106 (16.5, 12) -> (16.5, 19) construction
  line L107 (19.5, 12) -> (19.5, 19)
  line L108 (13.5, 19) -> (13.5, 12)
  arc A92 (13.5, 12) -> (19.5, 12) centre (16.5, 12) ccw
  arc A93 (19.5, 19) -> (13.5, 19) centre (16.5, 19) ccw
  line L109 (37.5, 43) -> (37.5, 50) construction
  line L110 (34.5, 43) -> (34.5, 50)
  line L111 (40.5, 50) -> (40.5, 43)
  arc A94 (34.5, 43) -> (40.5, 43) centre (37.5, 43) ccw
  arc A95 (40.5, 50) -> (34.5, 50) centre (37.5, 50) ccw
  point P0 (0, 0)
  point P1 (-40.5, -46.5)
  point P2 (-19.5, -15.5)
  point P3 (-97.5, -46.5)
  point P4 (-76.5, -15.5)
  point P5 (-97.5, 46.5)
  point P6 (-76.5, 15.5)
  point P7 (-19.5, 15.5)
  point P8 (-40.5, 46.5)
  point P9 (94.5, -46.5)
  point P10 (73.5, -15.5)
  point P11 (73.5, 15.5)
  point P12 (94.5, 46.5)
  point P13 (37.5, -46.5)
  point P14 (16.5, -15.5)
  point P15 (16.5, 15.5)
  point P16 (37.5, 46.5)
  point P17 (73.5, 9)
  point P18 (73.5, -22)
  point P19 (16.5, -22)
  point P20 (16.5, 9)
  point P21 (-40.5, 40)
  point P22 (-19.5, 22)
  point P23 (-40.5, -53)
  point P24 (-97.5, -53)
  constraints: 128 end point, 64 point on circle, 64 tangent, 32 centre point, 26 parallel, 16 midpoint, 1 vertical
extrude "Extrusion11" cut sketch "Sketch26" against normal blind 10 contours A3 L3 A2 A72 L77 A73 | A7 L7 A6 A75 L80 A74 | A11 L11 A10 A70 L74 A71 | A69 L71 A68 A13 L13 A12 | A64 L65 A65 A17 L17 A16 | A23 L23 A22 A66 L68 A67 | A27 L27 A26 A76 L83 A77 | A79 L86 A78 A29 L29 A28 | A35 L35 A34 A94 L110 A95 | A93 L107 A92 A37 L37 A36 | A91 L104 A90 A41 L41 A40 | A47 L47 A46 A88 L101 A89 | A51 L51 A50 A80 L90 A81 | A83 L92 A82 A53 L53 A52 | A85 L95 A84 A57 L57 A56 | A63 L63 A62 A86 L98 A87
hole "Hole20" at (-76.5, -70, 12.7) at (-19.5, -70, 12.7) at (16.5, -70, 12.7) at (73.5, -70, 12.7) direction (0, 1, 0) diameter 5.9436 depth 59 tip angle 118 taper from width 6.3893 to width 5.9591 over 6.886 thread size "1/16" designation "1/16 - 27 NPT" standard "NPT"
sketch "Sketch28" plane through (-117.5, 70, 0) normal (0, 1, 0) x (1, 0, 0)
  line L0 (0, 0) -> (0, -23.4) projected
  line L1 (235, 0) -> (0, 0) projected
  point P0 (117.5, 0)
  point P1 (20, -12.7)
  point P2 (41, -12.7)
  point P3 (77, -12.7)
  point P4 (98, -12.7)
  point P5 (134, -12.7)
  point P6 (155, -12.7)
  point P7 (191, -12.7)
  point P8 (212, -12.7)
  dimension "d545" = 20
  dimension "d546" = 21
  dimension "d547" = 12.7
  dimension "d550" = 57
  constraints: 1 horizontal, 1 horizontal alignment, 6 other
  measures "d545" distance from line of point (20, -12.7) L0
  measures "d546" distance of point (20, -12.7) point (41, -12.7)
  measures "d547" distance from line of L1 point (20, -12.7)
  measures "d550" distance of point (20, -12.7) point (77, -12.7)
hole "Hole21" at (-76.5, 70, 12.7) at (-19.5, 70, 12.7) at (16.5, 70, 12.7) at (73.5, 70, 12.7) direction (0, -1, 0) diameter 5.9436 depth 59 tip angle 118 taper from width 6.3893 to width 5.9591 over 6.886 thread size "1/16" designation "1/16 - 27 NPT" standard "NPT"
hole "Hole22" at (-40.5, 70, 12.7) at (37.5, 70, 12.7) at (94.5, 70, 12.7) at (-97.5, 70, 12.7) direction (0, -1, 0) diameter 5.9436 depth 28 tip angle 118 taper from width 6.3893 to width 5.9591 over 6.8859 thread size "1/16" designation "1/16 - 27 NPT" standard "NPT"
